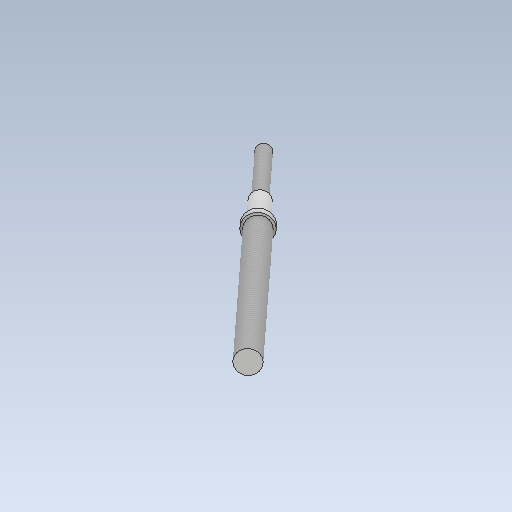
# Autodesk Inventor part: DEC_csavar
Saved by Autodesk Inventor 2021.4 (Build 254397000, 397)
## iProperties
Created: 2023-12-02
Part Number: DEC_csavar
Material: Generic
Document SubType Name: Modeling
Designer: vtoth
Density: 1 g/cm^3
Appearance: Default
Author: vtoth
Autodesk Inventor part; units mm, degrees
ref_plane "YZ Plane" through (0, 0, 0) normal (1, 0, 0) x (0, 1, 0)
ref_plane "XZ Plane" through (0, 0, 0) normal (0, 1, 0) x (-1, 0, 0)
ref_plane "XY Plane" through (0, 0, 0) normal (0, 0, 1) x (1, 0, 0)
derived "skeleton_1.ipt"
sketch "Sketch7" plane through (-58.4006, 79, 692.6521) normal (-0.0929708, 0.9906647, -0.099699) x (0.8216319, 0.1328926, 0.554311)
  line L0 (89.7407, 0) -> (4.4573, 19.497)
  line L1 (4.4573, 19.497) -> (0, 0)
  line L2 (93.0837, 14.6227) -> (89.7407, 0)
  point P0 (3.5658, 15.5976)
  point P1 (5.3487, 23.3964)
  point P2 (90.855, 4.8742)
  point P3 (88.6264, -4.8742)
ref_plane "Work Plane4" through (15.3332, 90.9259, 742.3963) normal (-0.0929708, 0.9906647, -0.099699) x (-0.6756317, -0.1363212, -0.7245263)
sketch "Sketch2" plane through (349.8021, 79.9658, 321.5937) normal (-0.0929708, 0.9906647, -0.099699) x (0.9922591, 0.0839069, -0.0915507)
  line L0 (-369.4849, -390.5704) -> (-423.3319, -321.622) projected
  line L1 (-373.4256, -393.648) -> (-431.8989, -318.7757)
  line L2 (-431.8989, -318.7757) -> (-432.6871, -319.3912)
  line L3 (-432.6871, -319.3912) -> (-434.5336, -317.0268)
  line L4 (-434.5336, -317.0268) -> (-432.9573, -315.7958)
  line L5 (-432.9573, -315.7958) -> (-443.421, -302.3975)
  line L6 (-443.421, -302.3975) -> (-442.6329, -301.782)
  line L7 (-442.6329, -301.782) -> (-464.1757, -274.1975)
  line L8 (-464.1757, -274.1975) -> (-461.8113, -272.351)
  line L9 (-461.8113, -272.351) -> (-369.4849, -390.5704)
  line L10 (-369.4849, -390.5704) -> (-373.4256, -393.648)
  point P0 (-365.5443, -387.4929)
  point P1 (-426.4844, -324.084)
  point P2 (-420.1794, -319.1599)
  point P3 (-423.3319, -321.622)
  dimension "d16" = 1
  dimension "d17" = 3
  dimension "d18" = 150
  dimension "d19" = 95
  dimension "d20" = 35
  dimension "d21" = 6
  constraints: 20 end point, 8 perpendicular, 4 point on line
  measures "d16" distance between parallel lines of L1 L3
  measures "d17" distance between parallel lines of L2 L4
  measures "d18" distance between parallel lines of L10 L8
  measures "d19" distance between parallel lines of L10 L2
  measures "d20" distance from line of L8.end L6
  measures "d21" diameter of L7 L0
revolve "Revolution1" add sketch "Sketch2" angle 360 about axis through (15.3332, 90.9259, 742.3963) along (-0.6756317, -0.1363212, -0.7245263)
thread "Thread1" size "M10x1.5" class "6g" standard "ISO Metric profile" full length
thread "Thread2" size "M6x1" class "6g" standard "ISO Metric profile" full length
body "Solid1"
